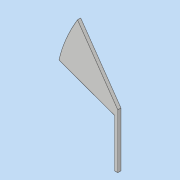
# Autodesk Inventor part: PropShroudSupport
Saved by Autodesk Inventor 2017 (Build 210142000, 142)
## iProperties
Created: 2017-03-05
Part Number: PropShroudSupport
Material: Generic
Document SubType Name: Modeling
Designer: techn
Density: 1 g/cm^3
Appearance: Default
Author: techn
Autodesk Inventor part; units mm, degrees
ref_plane "YZ Plane" through (0, 0, 0) normal (1, 0, 0) x (0, 1, 0)
ref_plane "XZ Plane" through (0, 0, 0) normal (0, 1, 0) x (-1, 0, 0)
ref_plane "XY Plane" through (0, 0, 0) normal (0, 0, 1) x (1, 0, 0)
sketch "Sketch1" plane through (0, 0, 0) normal (0, 0, 1) x (1, 0, 0)
  spline S0 degree 2 poles (0, 0) (-0.0954, 5.659) (4.0834, 12.7289) knots 0 0 0 1 1 1
  line L0 (0, 0) -> (-3.175, 0)
  line L1 (-3.175, 0) -> (11.43, 0)
  line L2 (11.43, 0) -> (11.43, -9.525)
  line L3 (11.43, -9.525) -> (12.065, -9.525)
  line L4 (12.065, -9.525) -> (12.065, 0)
  line L5 (11.43, 0) -> (0.4277, 4.0045)
  line L6 (12.065, 0) -> (12.065, 1.27)
  line L7 (12.065, 1.27) -> (4.0834, 12.7289)
  point P0 (0.7864, 5.4019)
  dimension "d0" = 4.0834
  dimension "d1" = 12.7289
  dimension "d2" = 7.327
  dimension "d3" = 3.297
  dimension "d4" = 3.175
  dimension "d5" = 14.605
  dimension "d6" = 9.525
  dimension "d7" = 0.635
  dimension "d8" = 20
  dimension "d11" = 1.27
  constraints: 16 end point, 2 horizontal, 2 perpendicular, 2 vertical, 1 coincident, 4 other
  measures "d0" horizontal distance of L7.end L0.start
  measures "d1" vertical distance of L0.start L7.end
  measures "d2" vertical distance of L7.end point (0.786, 5.402)
  measures "d3" horizontal distance of point (0.786, 5.402) L7.end
  measures "d4" distance of L0.start L0.end
  measures "d5" distance of L0.end L1.end
  measures "d6" distance of L1.end L2.end
  measures "d7" distance of L2.end L3.end
  measures "d8" angle of L1 L5
  measures "d11" distance of L4.end L6.end
extrude "Extrusion2" add sketch "Sketch1" along normal blind 0.635 contours S0 L7 L6 L4 L3 L2 L5
body "Solid2"
